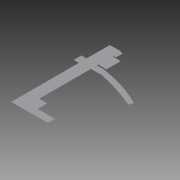
# Autodesk Inventor part: LabVIEWM0.5
Saved by Autodesk Inventor 2013 SP2 (Build 170200200, 200)
## iProperties
Created: 2014-11-17
Part Number: LabVIEWM0.5
Material: 常规
Document SubType Name: Modeling
Designer: 振胜
Density: 1 g/cm^3
Author: 振胜
Autodesk Inventor part; units mm, degrees
ref_plane "YZ Plane" through (0, 0, 0) normal (1, 0, 0) x (0, 1, 0)
ref_plane "工作平面1" through (0, 0, 42) normal (0, 0, 1) x (1, 0, 0)
sketch "草图1" plane through (0, 0, 42) normal (0, 0, 1) x (1, 0, 0)
  line L0 (0, 0) -> (60, 0)
  line L1 (60, 0) -> (60, -1169.8)
  line L2 (60, -1169.8) -> (0, -1169.8)
  line L3 (0, -1169.8) -> (0, 0)
  line L4 (0, -80.6) -> (60, -80.6)
  line L5 (0, -191.9) -> (60, -191.9)
  line L6 (0, -276.5) -> (60, -276.5)
  line L7 (0, -335.9) -> (60, -335.9)
  line L8 (0, -420.6) -> (60, -420.6)
  line L9 (0, -550.6) -> (60, -550.6)
  line L10 (0, -677.8) -> (60, -677.8)
  line L11 (0, -782.9) -> (60, -782.9)
  line L12 (0, -839.5) -> (60, -839.5)
  line L13 (0, -923.6) -> (60, -923.6)
  line L14 (0, -1007.7) -> (60, -1007.7)
  line L15 (0, -1091.2) -> (60, -1091.2)
  line L16 (60, 0) -> (118.4, 0)
  line L17 (118.4, 0) -> (118.4, -23.7)
  line L18 (118.4, -23.7) -> (83.4, -23.7)
  line L19 (83.4, -23.7) -> (83.4, -79.7)
  line L20 (83.4, -79.7) -> (118.4, -79.7)
  line L21 (118.4, -79.7) -> (118.4, -137.6)
  line L22 (118.4, -137.6) -> (83.4, -137.6)
  line L23 (83.4, -137.6) -> (83.4, -276.5)
  line L24 (83.4, -276.5) -> (142.9, -276.5)
  line L25 (142.9, -276.5) -> (142.9, -379.5)
  line L26 (83.4, -276.5) -> (83.4, -379.5)
  line L27 (83.4, -379.5) -> (142.9, -379.5)
  line L28 (142.9, -379.5) -> (142.9, -463)
  line L29 (142.9, -463) -> (83.4, -463)
  line L30 (83.4, -463) -> (83.4, -379.5)
  line L31 (142.9, -463) -> (142.9, -566.2)
  line L32 (142.9, -566.2) -> (83.4, -566.2)
  line L33 (83.4, -566.2) -> (83.4, -463)
  line L34 (142.9, -566.2) -> (146.7, -566.2)
  line L35 (146.7, -566.2) -> (146.7, -616.2)
  line L36 (146.7, -616.2) -> (192.5, -616.2)
  line L37 (192.5, -616.2) -> (192.5, -673.2)
  line L38 (192.5, -616.2) -> (342.5, -616.2)
  line L39 (342.5, -616.2) -> (342.5, -673.2)
  line L40 (342.5, -673.2) -> (143.4, -673.2)
  line L41 (143.4, -673.2) -> (83.4, -673.2)
  line L42 (83.4, -673.2) -> (83.4, -1092.3)
  line L43 (83.4, -1092.3) -> (143.4, -1092.3)
  line L44 (143.4, -1092.3) -> (143.4, -673.2)
  line L45 (83.4, -754.3) -> (143.4, -754.3)
  line L46 (143.4, -837.8) -> (83.4, -837.8)
  line L47 (83.4, -893.6) -> (143.4, -893.6)
  line L48 (143.4, -978.3) -> (83.4, -978.3)
  line L49 (60, -1169.8) -> (188.1, -1169.8)
  line L50 (188.1, -1169.8) -> (188.1, -1092.3)
  line L51 (188.1, -1092.3) -> (143.4, -1092.3)
  line L52 (83.4, -1092.3) -> (83.4, -1117.3)
  line L53 (83.4, -1117.3) -> (188.1, -1117.3)
  line L54 (98.6, -1092.3) -> (98.6, -1117.3)
  line L55 (114.5, -1092.3) -> (114.5, -1117.3)
  line L56 (143.4, -1092.3) -> (143.4, -1117.3)
  line L57 (166.2, -1092.3) -> (166.2, -1117.3)
  line L58 (188.1, -1163.6) -> (336, -1163.6)
  line L59 (188.1, -1137.1) -> (336, -1137.1)
  line L60 (336, -1137.1) -> (336, -1163.6)
  line L61 (342.5, -616.2) -> (398.5, -616.2)
  line L62 (342.5, -673.2) -> (393, -673.2)
  line L63 (393, -673.2) -> (393, -1136.7)
  line L64 (393, -1136.7) -> (393, -1141.7)
  line L65 (393, -1136.7) -> (336, -1137.1)
  line L66 (336, -1163.6) -> (393, -1163.6)
  line L67 (393, -1163.6) -> (393, -1158.6)
  line L68 (393, -1163.6) -> (393, -1188.1)
  line L69 (393, -1188.1) -> (417, -1188.1)
  line L70 (417, -1188.1) -> (542.5, -1188.1)
  line L71 (542.5, -1188.1) -> (542.5, -1127.7)
  line L72 (417, -1188.1) -> (417, -1127.7)
  line L73 (417, -1127.7) -> (542.5, -1127.7)
  line L74 (542.5, -1127.7) -> (542.5, -896.8)
  line L75 (542.5, -896.8) -> (542.5, -786.2)
  line L76 (542.5, -786.2) -> (542.5, -673.6)
  line L77 (542.5, -673.6) -> (393, -673.2)
  line L78 (417, -1127.7) -> (417, -896.8)
  line L79 (417, -896.8) -> (542.5, -896.8)
  line L80 (417, -896.8) -> (417.2959, -786.2)
  line L81 (417.2959, -786.2) -> (542.5, -786.2)
  line L82 (417.2959, -786.2) -> (417.5981, -673.2658)
  line L83 (398.5, -499.2) -> (398.5, -384.2)
  line L84 (398.5, -616.2) -> (398.5, -499.2)
  line L85 (398.5, -616.2) -> (458.5, -616.2)
  line L86 (458.5, -616.2) -> (458.5, -384.2)
  line L87 (458.5, -384.2) -> (398.5, -384.2)
  line L88 (398.5, -499.2) -> (458.5, -499.2)
  line L89 (398.5, -441.7) -> (458.5, -441.7)
  line L90 (458.5, -384.2) -> (458.5, -354.2)
  line L91 (458.5, -354.2) -> (482.5, -369.2)
  line L92 (482.5, -369.2) -> (482.5, -384.2)
  line L93 (482.5, -384.2) -> (542.5, -384.2)
  line L94 (542.5, -384.2) -> (542.5, -413.6)
  line L95 (542.5, -413.6) -> (542.5, -443.7)
  line L96 (542.5, -443.7) -> (542.5, -498.7)
  line L97 (542.5, -498.7) -> (542.5, -616.2)
  line L98 (542.5, -413.6) -> (501.5, -413.6)
  line L99 (542.5, -443.7) -> (482.5, -443.7)
  line L100 (542.5, -616.2) -> (482.5, -616.2)
  line L101 (542.5, -498.7) -> (482.5, -498.7)
  line L102 (482.5, -410.1) -> (501.5, -410.1)
  line L103 (501.5, -410.1) -> (501.5, -423.1)
  line L104 (501.5, -423.1) -> (482.5, -423.1)
  line L105 (482.5, -384.2) -> (482.5, -410.1)
  line L106 (482.5, -423.1) -> (482.5, -616.2)
  line L107 (542.5, -616.2) -> (727.5, -616.2)
  line L108 (727.5, -616.2) -> (727.5, -673.6)
  line L109 (727.5, -673.6) -> (542.5, -673.6)
  line L110 (578, -673.6) -> (578, -726.6)
  line L111 (578, -726.6) -> (605, -726.6)
  line L112 (605, -726.6) -> (605, -673.6)
  line L113 (727.5, -673.6) -> (727.5, -726.6)
  line L114 (727.5, -726.6) -> (700.5, -726.6)
  line L115 (700.5, -726.6) -> (700.5, -673.6)
  line L116 (442.5, -384.2) -> (442.5, -354.2)
  line L117 (442.5, -354.2) -> (458.5, -354.2)
  line L118 (398.5, -384.2) -> (384.5, -384.2)
  line L119 (384.5, -384.2) -> (384.5, -354.2)
  line L120 (384.5, -354.2) -> (400.5, -354.2)
  line L121 (400.5, -354.2) -> (400.5, -384.2)
  line L122 (727.5, -616.2) -> (765.5, -616.2)
  line L123 (765.5, -616.2) -> (825.5, -616.2)
  line L124 (765.5, -616.2) -> (765.5, -504.2)
  line L125 (765.5, -504.2) -> (765.5, -444.2)
  line L126 (765.5, -444.2) -> (825.5, -444.2)
  line L127 (825.5, -444.2) -> (825.5, -504.2)
  line L128 (825.5, -504.2) -> (825.5, -616.2)
  line L129 (825.5, -504.2) -> (765.5, -504.2)
  line L130 (825.5, -444.2) -> (849.2, -444.2)
  line L131 (849.2, -444.2) -> (849.2, -450.2)
  line L132 (849.2, -450.2) -> (868.2, -450.2)
  line L133 (868.2, -450.2) -> (868.2, -502.2)
  line L134 (868.2, -502.2) -> (849.2, -502.2)
  line L135 (849.2, -502.2) -> (849.2, -450.2)
  line L136 (849.2, -502.2) -> (849.2, -506.7)
  line L137 (849.2, -506.7) -> (909.2, -506.7)
  line L138 (909.2, -506.7) -> (909.2, -613.1)
  line L139 (909.2, -613.1) -> (849.2, -613.1)
  line L140 (849.2, -613.1) -> (849.2, -506.7)
  line L141 (727.5, -673.6) -> (765.5, -673.6)
  line L142 (765.5, -673.6) -> (765.5, -786.6)
  line L143 (765.5, -786.6) -> (825.5, -786.6)
  line L144 (825.5, -786.6) -> (825.5, -673.6)
  line L145 (825.5, -673.6) -> (765.5, -673.6)
  line L146 (765.5, -786.6) -> (765.5, -897.6)
  line L147 (765.5, -897.6) -> (825.5, -897.6)
  line L148 (825.5, -897.6) -> (825.5, -786.6)
  line L149 (765.5, -897.6) -> (765.5, -1008.6)
  line L150 (765.5, -1008.6) -> (825.5, -1008.6)
  line L151 (825.5, -1008.6) -> (825.5, -897.6)
  line L152 (765.5, -1008.6) -> (765.5, -1125.1)
  line L153 (765.5, -1125.1) -> (825.5, -1125.1)
  line L154 (825.5, -1125.1) -> (825.5, -1008.6)
  line L155 (765.5, -1125.1) -> (765.5, -1174.6)
  line L156 (765.5, -1174.6) -> (825.5, -1174.6)
  line L157 (825.5, -1174.6) -> (825.5, -1125.1)
  line L158 (825.5, -1174.6) -> (849.2, -1174.6)
  line L159 (849.2, -613.1) -> (849.2, -623.1)
  line L160 (849.2, -623.1) -> (916.2, -623.1)
  line L161 (916.2, -623.1) -> (916.2, -626.6)
  line L162 (849.2, -623.1) -> (849.2, -668.1)
  line L163 (849.2, -668.1) -> (916.2, -668.1)
  line L164 (916.2, -668.1) -> (916.2, -664.6)
  line L165 (849.2, -668.1) -> (849.2, -681.1)
  line L166 (849.2, -681.1) -> (849.2, -1050.1)
  line L167 (849.2, -1050.1) -> (909.2, -1050.1)
  line L168 (909.2, -1050.1) -> (909.2, -1091.6)
  line L169 (909.2, -1091.6) -> (909.2, -1121.1)
  line L170 (909.2, -1121.1) -> (849.2, -1121.1)
  line L171 (849.2, -1121.1) -> (849.2, -1050.1)
  line L172 (909.2, -1091.6) -> (849.2, -1091.6)
  line L173 (849.2, -1174.6) -> (849.2, -1121.1)
  line L174 (849.2, -1174.6) -> (1031.2, -1174.6)
  line L175 (1031.2, -1121.1) -> (909.2, -1121.1)
  line L176 (1031.2, -1121.1) -> (1031.2, -1174.6)
  line L177 (916.2, -626.6) -> (1226.4, -727) construction
  arc A0 (1226.4, -727) -> (916.2, -626.6) centre (761.993, -1632.4479) ccw
  line L178 (916.2, -664.6) -> (1213.4, -757.7) construction
  arc A1 (1213.4, -757.7) -> (916.2, -664.6) centre (605.6007, -2177.0365) ccw
  line L179 (1226.4, -727) -> (1213.4, -757.7)
  line L180 (1226.4, -727) -> (1239.7468, -733.8456)
  line L181 (1213.4, -757.7) -> (1226.7468, -764.5456)
  line L182 (1239.7468, -733.8456) -> (1237.0998, -739.0064)
  line L183 (1226.7468, -764.5456) -> (1229.3938, -759.3849)
  dimension "d1" = 60
  dimension "d2" = 80.6
  dimension "d3" = 111.3
  dimension "d4" = 84.6
  dimension "d5" = 59.4
  dimension "d6" = 84.7
  dimension "d7" = 130
  dimension "d8" = 127.2
  dimension "d9" = 105.1
  dimension "d10" = 56.6
  dimension "d11" = 84.1
  dimension "d12" = 84.1
  dimension "d13" = 83.5
  dimension "d14" = 78.6
  dimension "d15" = 58.4
  dimension "d16" = 23.7
  dimension "d17" = 35
  dimension "d18" = 56
  dimension "d19" = 57.9
  dimension "d20" = 35
  dimension "d21" = 138.9
  dimension "d22" = 59.5
  dimension "d23" = 103
  dimension "d24" = 83.5
  dimension "d25" = 103.2
  dimension "d26" = 59.5
  dimension "d27" = 3.8
  dimension "d28" = 50
  dimension "d29" = 45.8
  dimension "d30" = 57
  dimension "d31" = 150
  dimension "d32" = 57
  dimension "d33" = 199.1
  dimension "d34" = 60
  dimension "d36" = 81.1
  dimension "d37" = 83.5
  dimension "d38" = 55.8
  dimension "d39" = 84.7
  dimension "d40" = 114
  dimension "d41" = 128.1
  dimension "d42" = 25
  dimension "d43" = 15.2
  dimension "d44" = 15.9
  dimension "d45" = 28.9
  dimension "d46" = 22.8
  dimension "d47" = 21.9
  dimension "d48" = 147.9
  dimension "d49" = 6.2
  dimension "d50" = 26.5
  dimension "d51" = 56
  dimension "d52" = 50.5
  dimension "d53" = 463.5
  dimension "d54" = 5
  dimension "d55" = 5
  dimension "d56" = 24.5
  dimension "d57" = 24
  dimension "d58" = 125.5
  dimension "d59" = 60.4
  dimension "d60" = 230.9
  dimension "d61" = 110.6
  dimension "d62" = 112.6
  dimension "d64" = 117
  dimension "d65" = 115
  dimension "d66" = 60
  constraints: 364 end point, 94 perpendicular, 39 parallel, 37 point on line, 19 horizontal, 14 collinear, 7 vertical, 4 point on circle, 2 centre point, 1 horizontal alignment, 1 midpoint, 1 tangent, 1 vertical alignment, 30 other
  measures "d1" distance of L0.start L0.end
  measures "d2" distance between parallel lines of L4 L0
  measures "d3" distance between parallel lines of L5 L4
  measures "d4" distance between parallel lines of L6 L5
  measures "d5" distance between parallel lines of L7 L6
  measures "d6" distance between parallel lines of L8 L7
  measures "d7" distance between parallel lines of L9 L8
  measures "d8" distance between parallel lines of L10 L9
  measures "d9" distance between parallel lines of L11 L10
  measures "d10" distance between parallel lines of L12 L11
  measures "d11" distance between parallel lines of L13 L12
  measures "d12" distance between parallel lines of L14 L13
  measures "d13" distance between parallel lines of L15 L14
  measures "d14" distance between parallel lines of L2 L15
  measures "d15" distance of L0.end L16.end
  measures "d16" distance of L16.end L17.end
  measures "d17" distance of L17.end L18.end
  measures "d18" distance of L18.end L19.end
  measures "d19" distance of L20.end L21.end
  measures "d20" distance of L21.end L22.end
  measures "d21" distance of L22.end L23.end
  measures "d22" distance of L23.end L24.end
  measures "d23" distance of L24.end L25.end
  measures "d24" distance of L25.end L28.end
  measures "d25" distance of L28.end L31.end
  measures "d26" distance of L31.end L32.end
  measures "d27" distance of L31.end L34.end
  measures "d28" distance of L34.end L35.end
  measures "d29" distance of L35.end L36.end
  measures "d30" distance of L36.end L37.end
  measures "d31" distance of L36.end L38.end
  measures "d32" distance of L38.end L39.end
  measures "d33" distance of L39.end L40.end
  measures "d34" distance of L40.end L41.end
  measures "d36" distance between parallel lines of L45 L41
  measures "d37" distance between parallel lines of L46 L45
  measures "d38" distance between parallel lines of L47 L46
  measures "d39" distance between parallel lines of L48 L47
  measures "d40" distance between parallel lines of L43 L48
  measures "d41" distance of L2.start L49.end
  measures "d42" distance between parallel lines of L53 L51
  measures "d43" distance between parallel lines of L54 L52
  measures "d44" distance between parallel lines of L55 L54
  measures "d45" distance between parallel lines of L56 L55
  measures "d46" distance between parallel lines of L57 L56
  measures "d47" distance between parallel lines of L50 L57
  measures "d48" distance of L58.start L58.end
  measures "d49" distance between parallel lines of L49 L58
  measures "d50" distance between parallel lines of L58 L59
  measures "d51" distance of L38.end L61.end
  measures "d52" distance of L39.end L62.end
  measures "d53" distance of L62.end L63.end
  measures "d54" distance of L63.end L64.end
  measures "d55" distance of L66.end L67.end
  measures "d56" distance of L66.end L68.end
  measures "d57" distance of L68.end L69.end
  measures "d58" distance of L69.end L70.end
  measures "d59" distance of L70.end L71.end
  measures "d60" distance of L71.end L74.end
  measures "d61" distance of L74.end L75.end
  measures "d62" distance of L75.end L76.end
  measures "d64" distance of L61.end L83.start
  measures "d65" distance of L83.start L83.end
  measures "d66" distance of L61.end L85.end
extrude "拉伸1" add sketch "草图1" against normal blind 1 contours L108 L122 L123 L128 L127 L130 L131 L135 L136 L140 L159 L162 L165 L166 L171 L173 L158 L157 L154 L151 L148 L144 L145 L141 | L145 L144 L143 L142 | L124 L129 L128 L123 | L143 L148 L147 L146 | L125 L126 L127 L129 | L147 L151 L150 L149 | L150 L154 L153 L152 | L153 L157 L156 L155 | L132 L133 L134 L135 | L173 L170 L175 L176 L174 | L137 L138 L139 L140 | L171 L172 L169 L170 | L171 L167 L168 L172 | L160 L161 A0 L179 A1 L164 L163 L162
sketch "草图2" plane through (765.5, -1174.6, 42) normal (0, -1, 0) x (1, 0, 0)
  line L0 (265.7, 0) -> (265.7, -1) construction
  line L1 (265.7, -0.5) -> (280.7, 7)
  line L2 (265.7, -0.5) -> (265.7, -0.1)
  line L3 (265.7, -0.1) -> (280.7, 7.4)
  line L4 (280.7, 7.4) -> (280.7, 7)
  point P0 (-765.5, -42)
  dimension "d135" = 7.5
  dimension "d137" = 15
  dimension "d138" = 0.4
  constraints: 8 end point, 1 midpoint, 1 parallel, 1 point on line, 1 vertical
  measures "d135" vertical distance of L1.start L1.end
  measures "d137" horizontal distance of L1.start L1.end
  measures "d138" distance of L1.start L2.end
extrude "拉伸2" add sketch "草图2" against normal up to surface (53.5 mm away)
ref_plane "工作平面2" through (1226.4, -727, 42) normal (0.3899335, 0.920843, 0) x (-0.920843, 0.3899335, 0)
sketch "草图3" plane through (1226.4, -727, 42) normal (0.3899335, 0.920843, 0) x (-0.920843, 0.3899335, 0)
  line L0 (0, 0) -> (0, -1) construction
  line L1 (0, -0.5) -> (-15, 7)
  line L2 (0, -0.5) -> (0, -0.1)
  line L3 (0, -0.1) -> (-15, 7.4)
  line L4 (-15, 7.4) -> (-15, 7)
  point P0 (1412.8035, -42)
  dimension "d141" = 7.5
  dimension "d144" = 15
  dimension "d145" = 0.4
  constraints: 8 end point, 1 midpoint, 1 parallel, 1 point on line, 1 vertical
  measures "d141" vertical distance of L1.start L1.end
  measures "d144" horizontal distance of L1.start L1.end
  measures "d145" distance of L1.start L2.end
extrude "拉伸3" add sketch "草图3" against normal blind 33.4
